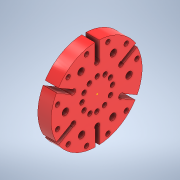
# Autodesk Inventor part: hw10
Saved by Autodesk Inventor 2021 (Build 250183000, 183)
## iProperties
Created: 2022-04-30
Part Number: hw10
Material: Generic
Document SubType Name: Modeling
Designer: authe
Density: 1 g/cm^3
Appearance: Light Red
Author: authe
Autodesk Inventor part; units mm, degrees
ref_plane "YZ Plane" through (0, 0, 0) normal (1, 0, 0) x (0, 1, 0)
ref_plane "XZ Plane" through (0, 0, 0) normal (0, 1, 0) x (-1, 0, 0)
ref_plane "XY Plane" through (0, 0, 0) normal (0, 0, 1) x (1, 0, 0)
sketch "Sketch2" plane through (0, 0, 0) normal (1, 0, 0) x (0, 1, 0)
  circle A0 centre (29.9437, -8.0234) radius 1.75
  circle A1 centre (21.9203, -21.9203) radius 1.75
  circle A2 centre (20.6241, -12.1945) radius 2.5
  circle A3 centre (9.8159, -5.9548) radius 1.75
  arc A4 (9.75, 0) -> (13.25, 0) centre (11.5, 0) ccw
  arc A5 (6.625, -11.4748) -> (4.875, -8.4437) centre (5.75, -9.9593) ccw
  arc A6 (4.875, 8.4437) -> (6.625, 11.4748) centre (5.75, 9.9593) ccw
  circle A7 centre (21.9203, 21.9203) radius 1.75
  circle A8 centre (9.8159, 5.9548) radius 1.75
  arc A9 (13.25, 0) -> (9.75, 0) centre (11.5, 0) ccw
  circle A10 centre (20.659, 12.215) radius 2.5
  circle A11 centre (29.9437, 8.0234) radius 1.75
  arc A12 (-6.625, -11.4748) -> (-4.875, -8.4437) centre (-5.75, -9.9593) ccw
  circle A13 centre (0.2491, -11.4783) radius 1.75
  arc A14 (4.875, -8.4437) -> (6.625, -11.4748) centre (5.75, -9.9593) ccw
  circle A15 centre (0.2491, -23.9987) radius 2.5
  circle A16 centre (8.0234, -29.9437) radius 1.75
  circle A17 centre (-29.9437, 8.0234) radius 1.75
  arc A18 (-20.67, 27.7987) -> (-34.0375, 2.54) centre (-0.0705, 0.7304) ccw
  circle A19 centre (-21.9203, 21.9203) radius 1.75
  circle A20 centre (-20.908, 11.7837) radius 2.5
  circle A21 centre (-8.0234, 29.9437) radius 1.75
  circle A22 centre (0.2491, 23.9987) radius 2.5
  circle A23 centre (8.0234, 29.9437) radius 1.75
  circle A24 centre (-10.065, 5.5234) radius 1.75
  arc A25 (-6.625, 11.4748) -> (-4.875, 8.4437) centre (-5.75, 9.9593) ccw
  arc A26 (-9.577, 0.2829) -> (-13.077, 0.2829) centre (-11.327, 0.2829) ccw
  arc A27 (-4.875, 8.4437) -> (-6.625, 11.4748) centre (-5.75, 9.9593) ccw
  circle A28 centre (0.2491, 11.4783) radius 1.75
  arc A29 (6.625, 11.4748) -> (4.875, 8.4437) centre (5.75, 9.9593) ccw
  circle A30 centre (-10.065, -5.5234) radius 1.75
  arc A31 (-13.077, 0.2829) -> (-9.577, 0.2829) centre (-11.327, 0.2829) ccw
  circle A32 centre (-29.9437, -8.0234) radius 1.75
  circle A33 centre (-20.908, -11.7837) radius 2.5
  arc A34 (-4.875, -8.4437) -> (-6.625, -11.4748) centre (-5.75, -9.9593) ccw
  circle A35 centre (-21.9203, -21.9203) radius 1.75
  circle A36 centre (-0.0705, 0.7304) radius 11.5
  circle A37 centre (-0.0567, -0.0164) radius 16
  circle A38 centre (20.8777, 0.0604) radius 2
  circle A39 centre (10.3614, 18.1796) radius 2
  circle A40 centre (-10.5884, 18.1317) radius 2
  circle A41 centre (-21.0219, -0.0352) radius 2
  circle A42 centre (-10.5055, -18.1543) radius 2
  circle A43 centre (10.4442, -18.1065) radius 2
  line L0 (22.1372, 1.614) -> (33.5016, 1.614)
  line L1 (33.8933, -1.4213) -> (22.221, -1.4213)
  circle A44 centre (-0.0721, 0.0126) radius 21
  circle A45 centre (10.3614, 18.1796) radius 2
  line L2 (18.1524, 28.7106) -> (12.3162, 18.602)
  line L3 (9.6458, 20.0472) -> (15.3279, 29.889)
  circle A46 centre (-10.5884, 18.1317) radius 2
  line L4 (-15.813, 30.1445) -> (-9.9768, 20.0359)
  line L5 (-12.5636, 18.4458) -> (-18.2458, 28.2876)
  circle A47 centre (-21.0219, -0.0352) radius 2
  line L6 (-34.0375, 1.4465) -> (-22.3652, 1.4465)
  line L7 (-22.2814, -1.5888) -> (-33.6458, -1.5888)
  circle A48 centre (-10.5055, -18.1543) radius 2
  line L8 (-18.2966, -28.6853) -> (-12.4604, -18.5768)
  line L9 (-9.7899, -20.0219) -> (-15.4721, -29.8638)
  circle A49 centre (10.4442, -18.1065) radius 2
  line L10 (15.6688, -30.1192) -> (9.8327, -20.0107)
  line L11 (12.4194, -18.4206) -> (18.1016, -28.2624)
  line L12 (18.4756, 29.187) -> (19.0144, 28.8293)
  line L13 (-34.0375, 2.54) -> (-34.0375, 1.4465)
  arc A50 (-30.896, 15.1154) -> (-31.286, 14.2919) centre (-0.0721, 0.0126) ccw
  arc A51 (18.1835, -28.6656) -> (33.8029, -2.8495) centre (-0.0721, 0.0126) ccw
  arc A52 (-15.7518, -30.1511) -> (15.6688, -30.1192) centre (-0.0721, 0.0126) ccw
  arc A53 (-34.03, -1.5888) -> (-18.2966, -28.6853) centre (-0.0721, 0.0126) ccw
  line L14 (-31.2555, 14.3144) -> (-31.286, 14.2919)
  line L15 (-18.2458, 28.2876) -> (-18.7494, 29.1599)
  line L16 (-15.813, 30.1445) -> (-16.1409, 30.7124)
  arc A54 (16.0144, 30.7046) -> (-16.1409, 30.7124) centre (-0.0705, 0.7304) ccw
  arc A55 (-18.7494, 29.1599) -> (-30.896, 15.1154) centre (-0.0705, 0.7304) ccw
  line L17 (15.3279, 29.889) -> (16.0144, 30.7046)
  arc A56 (33.4181, -5.8277) -> (33.8933, -1.4213) centre (-0.0721, 0.0126) ccw
  line L18 (-15.4721, -29.8638) -> (-15.7518, -30.1511)
  line L19 (18.1524, 28.7106) -> (18.4708, 29.1902)
  arc A57 (34.4668, 1.614) -> (18.4708, 29.1902) centre (-0.0572, 0.0153) ccw
  line L20 (33.5016, 1.614) -> (34.4668, 1.614)
  arc A58 (18.5858, -29.1011) -> (34.4864, -1.4213) centre (-0.0572, 0.0153) ccw
  line L21 (12.4194, -18.4206) -> (18.5858, -29.1011)
  line L22 (22.221, -1.4213) -> (34.4864, -1.4213)
  line L23 (-33.6458, -1.5888) -> (-34.03, -1.5888)
  circle A59 centre (-7.6237, -27.9702) radius 1.75
  point P0 (13.25, 0)
  dimension "d1" = 1.75
  dimension "d2" = 5
  dimension "d8" = 3
  dimension "d9" = 23
  dimension "d11" = 32
  dimension "d18" = 360
  dimension "d23" = 42
  dimension "d26" = 360
  constraints: 60 centre point, 57 point on circle, 48 end point, 29 equal radius, 15 coincident, 4 horizontal, 4 point on line, 2 collinear, 1 perpendicular, 1 vertical, 62 other
  measures "d1" radius of A4
  measures "d2" diameter of A15
  measures "d8" horizontal distance of L17.end L12.end
  measures "d9" diameter of A36
  measures "d11" diameter of A37
  measures "d23" diameter of A44
extrude "Extrusion1" add sketch "Sketch2" along normal mid plane 10 contours A3 A36 A5 A14 A13 A12 A34 A30 A31 A26 A24 A25 A27 A28 A29 A6 A8 A9 A4 | A55 L15 L5 A40 A44 A41 L6 L13 A18 | A18 L14 A50 | L4 L16 A54 L17 L3 A39 A44 A40 | A40 A44 A39 A38 A43 A42 A41 | A41 A44 A42 L8 A53 L23 L7 | A39 L2 L19 A57 L20 L0 A38 A44 | A44 A43 L10 A52 L18 L9 A42 | A38 L1 A56 A51 L21 L11 A43 A44 | L22 A58 L21 A51 A56 | A37 | A59
sketch "Sketch9" plane through (5, 0, 0) normal (1, 0, 0) x (0, 0, -1)
  point P0 (0, 0)
body "Solid1"
